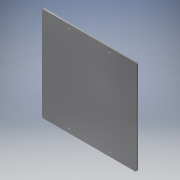
# Autodesk Inventor part: Stock Build Plate
Saved by Autodesk Inventor 2017 (Build 210142000, 142)
## iProperties
Created: 2017-03-10
Part Number: Stock Build Plate
Material: Generic
Document SubType Name: Modeling
Designer: gilef
Density: 1 g/cm^3
Appearance: Aluminum - Polished
Author: gilef
Autodesk Inventor part; units mm, degrees
ref_plane "YZ Plane" through (0, 0, 0) normal (1, 0, 0) x (0, 1, 0)
ref_plane "XZ Plane" through (0, 0, 0) normal (0, 1, 0) x (-1, 0, 0)
ref_plane "XY Plane" through (0, 0, 0) normal (0, 0, 1) x (1, 0, 0)
sketch "Sketch1" plane through (0, 0, 0) normal (0, 1, 0) x (-1, 0, 0)
  line L0 (-105, -105) -> (105, -105)
  line L1 (105, -105) -> (105, 105)
  line L2 (105, 105) -> (-105, 105)
  line L3 (-105, 105) -> (-105, -105)
  line L4 (-105, -105) -> (105, 105) construction
  line L5 (105, -105) -> (-105, 105) construction
  point P0 (0, 0)
  dimension "d0" = 210
  constraints: 12 end point, 2 midpoint, 2 parallel, 2 perpendicular, 1 horizontal
  measures "d0" distance of L0.end L1.end
extrude "Extrusion1" add sketch "Sketch1" along normal blind 3
sketch "Sketch2" plane through (0, 3, 0) normal (0, 1, 0) x (1, 0, 0)
  line L0 (45.25, 95) -> (-45.25, 95) construction
  line L1 (-45.25, 95) -> (-45.25, -95) construction
  line L2 (-45.25, -95) -> (45.25, -95) construction
  line L3 (45.25, -95) -> (45.25, 95) construction
  line L4 (45.25, 95) -> (-45.25, -95) construction
  line L5 (-45.25, 95) -> (45.25, -95) construction
  point P0 (0, 0)
  dimension "d3" = 190
  dimension "d4" = 90.5
  constraints: 12 end point, 2 midpoint, 2 parallel, 1 horizontal, 1 perpendicular
  measures "d3" distance of L2.end L0.start
  measures "d4" distance of L1.end L2.end
hole "Hole1" at (45.25, 3, 95) at (45.25, 3, -95) at (-45.25, 3, -95) at (-45.25, 3, 95) direction (0, -1, 0) diameter 3.5 end through all countersink diameter 7 countersink angle 90
fillet "Fillet1" radius 3 4 edges at (-105, 1.5, 105) (105, 1.5, 105) (105, 1.5, -105) (-105, 1.5, -105)
body "Solid1"
